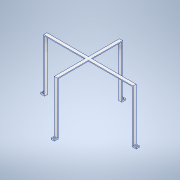
# Autodesk Inventor part: Soporte
Saved by Autodesk Inventor 2022.1 (Build 261234000, 234)
## iProperties
Created: 2021-10-03
Part Number: Soporte
Material: Aluminio 6061
Document SubType Name: Modeling
Designer: seb_0
Density: 2.7 g/cm^3
Appearance: Aluminio - Plano
Author: seb_0
Autodesk Inventor part; units mm, degrees
ref_plane "YZ Plane" through (0, 0, 0) normal (1, 0, 0) x (0, 1, 0)
ref_plane "XZ Plane" through (0, 0, 0) normal (0, 1, 0) x (-1, 0, 0)
ref_plane "XY Plane" through (0, 0, 0) normal (0, 0, 1) x (1, 0, 0)
sketch "Boceto1" plane through (0, 0, 0) normal (0, 1, 0) x (-1, 0, 0)
  line L0 (276.86, 5) -> (0, 5)
  line L1 (0, 5) -> (0, -5)
  line L2 (0, -5) -> (276.86, -5)
  line L3 (276.86, -5) -> (276.86, 5)
  line L4 (148.43, 100.33) -> (138.43, 100.33)
  line L5 (138.43, 100.33) -> (138.43, -100.33)
  line L6 (138.43, -100.33) -> (148.43, -100.33)
  line L7 (148.43, -100.33) -> (148.43, 100.33)
  line L8 (276.86, 0) -> (0, 0)
  point P0 (0, 0)
  point P1 (138.43, 0)
  point P2 (148.43, -5)
  point P3 (148.43, 5)
  point P4 (138.43, 5)
  point P5 (138.43, -5)
  dimension "d0" = 276.86
  dimension "d1" = 200.66
  dimension "d2" = 10
  dimension "d3" = 138.43
  constraints: 18 end point, 5 parallel, 4 midpoint, 3 perpendicular, 2 horizontal, 1 coincident
  measures "d0" distance of L0.start L0.end
  measures "d1" distance of L4.end L5.end
  measures "d2" distance of L2.end L0.start
  measures "d3" distance from line of point (0, 0) L5
extrude "Extrusión1" add sketch "Boceto1" along normal blind 2.5
sketch "Boceto2" plane through (-148.43, 0, 100.33) normal (0, 0, 1) x (1, 0, 0)
  line L0 (0, 0) -> (10, 0) projected
  line L1 (10, 0) -> (10, 2.5) projected
  line L2 (0, 2.5) -> (10, 2.5) projected
  line L3 (0, 0) -> (0, 2.5) projected
  line L4 (0, 0) -> (0, 2.5) projected
  line L5 (0, 0) -> (0, -165.1)
  line L6 (0, -165.1) -> (10, -165.1)
  line L7 (0, 0) -> (10, 0) projected
  line L8 (10, -165.1) -> (10, 0)
  point P0 (148.43, 0)
  dimension "d7" = 165.1
  constraints: 6 end point, 2 perpendicular, 1 vertical
  measures "d7" distance of L6.end L0.end
extrude "Extrusión2" add sketch "Boceto2" along normal blind 2.5
sketch "Boceto3" plane through (-138.43, 0, -100.33) normal (0, 0, -1) x (-1, 0, 0)
  line L0 (0, 0) -> (10, 0) projected
  line L1 (10, 0) -> (10, 2.5) projected
  line L2 (0, 2.5) -> (10, 2.5) projected
  line L3 (0, 0) -> (0, 2.5) projected
  line L4 (10, 0) -> (0, 0) projected
  line L5 (0, -165.1) -> (0, 0) projected
  line L6 (10, -165.1) -> (0, -165.1) projected
  line L7 (10, 0) -> (10, -165.1) projected
  point P0 (-138.43, 0)
extrude "Extrusión3" add sketch "Boceto3" along normal blind 2.5
sketch "Boceto4" plane through (0, 0, 5) normal (1, 0, 0) x (0, 0, -1)
  line L0 (0, 0) -> (10, 0) projected
  line L1 (10, 0) -> (10, 2.5) projected
  line L2 (0, 2.5) -> (10, 2.5) projected
  line L3 (0, 0) -> (0, 2.5) projected
  line L4 (0, 0) -> (0, -165.1)
  line L5 (0, -165.1) -> (10, -165.1)
  line L6 (10, -165.1) -> (10, 0)
  line L7 (105.33, 0) -> (105.33, -165.1) projected
  point P0 (5, 0)
  constraints: 6 end point, 2 perpendicular, 1 parallel, 1 vertical
extrude "Extrusión4" add sketch "Boceto4" along normal blind 2.5
sketch "Boceto5" plane through (-276.86, 0, -5) normal (-1, 0, 0) x (0, 0, 1)
  line L0 (0, 0) -> (10, 0) projected
  line L1 (10, 0) -> (10, 2.5) projected
  line L2 (0, 2.5) -> (10, 2.5) projected
  line L3 (0, 0) -> (0, 2.5) projected
  line L4 (10, 0) -> (0, 0) projected
  line L5 (0, -165.1) -> (0, 0) projected
  line L6 (10, -165.1) -> (0, -165.1) projected
  line L7 (10, 0) -> (10, -165.1) projected
  point P0 (5, 0)
extrude "Extrusión5" add sketch "Boceto5" along normal blind 2.5
sketch "Boceto6" plane through (-276.86, -165.1, -5) normal (0, -1, 0) x (1, 0, 0)
  line L0 (276.86, 10) -> (276.86, 0) projected
  line L1 (276.86, 0) -> (279.36, 0) projected
  line L2 (279.36, 10) -> (279.36, 0) projected
  line L3 (276.86, 10) -> (279.36, 10) projected
  line L4 (128.43, 105.33) -> (138.43, 105.33) projected
  line L5 (138.43, 105.33) -> (138.43, 107.83) projected
  line L6 (128.43, 107.83) -> (138.43, 107.83) projected
  line L7 (128.43, 105.33) -> (128.43, 107.83) projected
  line L8 (0, 0) -> (0, 10) projected
  line L9 (0, 10) -> (-2.5, 10) projected
  line L10 (-2.5, 0) -> (-2.5, 10) projected
  line L11 (0, 0) -> (-2.5, 0) projected
  line L12 (138.43, -95.33) -> (128.43, -95.33) projected
  line L13 (128.43, -95.33) -> (128.43, -97.83) projected
  line L14 (138.43, -97.83) -> (128.43, -97.83) projected
  line L15 (138.43, -95.33) -> (138.43, -97.83) projected
  line L16 (138.43, -97.83) -> (138.43, -107.83)
  line L17 (138.43, -107.83) -> (128.43, -107.83)
  line L18 (128.43, -97.83) -> (138.43, -97.83) projected
  line L19 (128.43, -107.83) -> (128.43, -97.83)
  line L20 (279.36, 0) -> (289.36, 0)
  line L21 (289.36, 0) -> (289.36, 10)
  line L22 (289.36, 10) -> (279.36, 10)
  line L23 (128.43, 10) -> (128.43, 107.83) projected
  line L24 (128.43, 107.83) -> (128.43, 117.83)
  line L25 (128.43, 117.83) -> (138.43, 117.83)
  line L26 (138.43, 117.83) -> (138.43, 107.83)
  line L27 (-2.5, 0) -> (-2.5, 10) projected
  line L28 (-2.5, 0) -> (-12.5, 0)
  line L29 (-12.5, 0) -> (-12.5, 10)
  line L30 (-12.5, 10) -> (-2.5, 10)
  circle A0 centre (-7.5, 5) radius 3
  circle A1 centre (133.43, 112.83) radius 3
  circle A2 centre (133.43, -102.83) radius 3
  circle A3 centre (284.36, 5) radius 3
  point P0 (276.86, 5)
  point P1 (-7.5, 10)
  point P2 (133.43, -107.83)
  dimension "d16" = 6
  dimension "d17" = 5
  dimension "d18" = 5
  dimension "d19" = 6
  dimension "d20" = 5
  dimension "d21" = 5
  dimension "d22" = 6
  dimension "d23" = 5
  dimension "d24" = 5
  dimension "d25" = 6
  dimension "d26" = 5
  dimension "d27" = 5
  constraints: 24 end point, 11 perpendicular, 4 centre point, 2 horizontal, 2 midpoint, 2 vertical, 1 parallel
  measures "d16" diameter of A0
  measures "d17" distance of point (-7.5, 10) A0.centre
  measures "d18" distance from line of L10 A0.centre
  measures "d19" diameter of A1
  measures "d20" distance from line of L24 A1.centre
  measures "d21" distance from line of L6 A1.centre
  measures "d22" diameter of A2
  measures "d23" distance of point (133.43, -107.83) A2.centre
  measures "d24" distance from line of L16 A2.centre
  measures "d25" diameter of A3
  measures "d26" distance from line of L22 A3.centre
  measures "d27" distance from line of L2 A3.centre
extrude "Extrusión6" add sketch "Boceto6" against normal blind 4 contours L22 L21 L20 L2 | L24 L25 L26 L6 | L28 L29 L30 L10 | L16 L17 L19 L14
